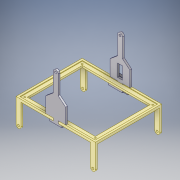
# Autodesk Inventor part: ControllerPCBHolder
Saved by Autodesk Inventor 2019.1 (Build 231200000, 200)
## iProperties
Created: 2018-09-15
Part Number: ControllerPCBHolder
Material: Generisch
Document SubType Name: Modeling
Designer: JochenAlt
Density: 1 g/cm^3
Appearance: Nylon 6
Author: JochenAlt
Autodesk Inventor part; units mm, degrees
ref_plane "YZ Plane" through (0, 0, 0) normal (1, 0, 0) x (0, 1, 0)
ref_plane "XZ Plane" through (0, 0, 0) normal (0, 1, 0) x (-1, 0, 0)
ref_plane "XY Plane" through (0, 0, 0) normal (0, 0, 1) x (1, 0, 0)
sketch "Skizze1" plane through (0, 0, 0) normal (0, 0, 1) x (1, 0, 0)
  line L0 (-61, 50.5) -> (61, 50.5)
  line L1 (61, 50.5) -> (61, -50.5)
  line L2 (61, -50.5) -> (-61, -50.5)
  line L3 (-61, -50.5) -> (-61, 50.5)
  line L4 (0, 70.7) -> (0, -70.7) construction
  line L5 (-85.4, 0) -> (85.4, 0) construction
  line L6 (-55, 44.5) -> (55, 44.5)
  line L7 (55, 44.5) -> (55, -44.5)
  line L8 (55, -44.5) -> (-55, -44.5)
  line L9 (-55, -44.5) -> (-55, 44.5)
  line L10 (-57.15, 46.36) -> (57.15, 46.36) construction
  line L11 (57.15, 46.36) -> (57.15, -46.36) construction
  line L12 (57.15, -46.36) -> (-57.15, -46.36) construction
  line L13 (-57.15, -46.36) -> (-57.15, 46.36) construction
  circle A0 centre (-57.15, 46.36) radius 1.25
  circle A1 centre (57.15, 46.36) radius 1.25
  circle A2 centre (-57.15, -46.36) radius 1.25
  circle A3 centre (57.15, -46.36) radius 1.25
  point P0 (0, 0)
  dimension "d0" = 122
  dimension "d1" = 101
  dimension "d4" = 6
  dimension "d5" = 6
  dimension "d6" = 2.5
  dimension "d7" = 114.3
  dimension "d8" = 92.72
  constraints: 24 end point, 6 parallel, 4 centre point, 4 coincident, 3 equal radius, 3 horizontal, 3 perpendicular, 6 other
  measures "d0" distance of L0.start L0.end
  measures "d1" distance of L0.end L1.end
  measures "d4" distance between parallel lines of L6 L0
  measures "d5" distance between parallel lines of L9 L3
  measures "d6" diameter of A0
  measures "d7" distance of L11.end L12.end
  measures "d8" distance of L10.end L11.end
extrude "Extrusion2" add sketch "Skizze1" along normal blind 3
sketch "Skizze2" plane through (0, 0, 0) normal (0, 1, 0) x (-1, 0, 0)
  arc A0 (56.1888, -34.75) -> (64.1888, -34.75) centre (60.1888, -34.75) ccw
  arc A1 (-64.1888, -34.75) -> (-56.1888, -34.75) centre (-60.1888, -34.75) ccw
  line L0 (0, -98.1) -> (0, 102.1) construction
  line L1 (-97.3, 0) -> (97.3, 0) construction
  circle A2 centre (60.1888, -34.75) radius 1.75
  circle A3 centre (-60.1888, -34.75) radius 1.75
  line L2 (64.1888, -34.75) -> (64.1888, 3)
  line L3 (56.1888, -34.75) -> (56.1888, 3)
  line L4 (-56.1888, -34.75) -> (-56.1888, 3)
  line L5 (-64.1888, -34.75) -> (-64.1888, 3)
  line L6 (-61, 3) -> (61, 3) construction
  line L7 (64.1888, 3) -> (56.1888, 3)
  line L8 (-64.1888, 3) -> (-56.1888, 3)
  circle A4 centre (0, 69.5) radius 1.75
  arc A5 (4, 69.5) -> (-4, 69.5) centre (0, 69.5) ccw
  line L9 (60.1888, -34.75) -> (0, 69.5) construction
  line L10 (4, 69.5) -> (4, 39)
  line L11 (-4, 0) -> (-4, 9)
  line L12 (61, 0) -> (-61, 0) projected
  circle A6 centre (0, 0) radius 69.5 construction
  line L13 (60.1888, -34.75) -> (-60.1888, -34.75) construction
  line L14 (0, 69.5) -> (-60.1888, -34.75) construction
  line L15 (-4.15, 0) -> (-4.15, 4)
  line L16 (-4.15, 4) -> (-4, 4)
  line L17 (4.15, 4) -> (4.15, 0)
  line L18 (55, 3) -> (-55, 3) construction
  line L19 (4.15, 0) -> (4, 0)
  line L20 (4, 0) -> (4, 0)
  line L21 (-4, 0) -> (-4.15, 0)
  line L22 (4, 0) -> (-4, 0)
  line L23 (4.15, 4) -> (16, 4)
  line L24 (16, 4) -> (16, 29)
  line L25 (16, 29) -> (4, 39)
  line L26 (4, 39) -> (-4, 39)
  line L27 (-4, 39) -> (-16, 29)
  line L28 (-16, 29) -> (-16, 4)
  line L29 (-16, 4) -> (-4.15, 4)
  line L30 (4, 29) -> (-4, 29)
  line L31 (4, 29) -> (4, 9)
  line L32 (-4, 29) -> (-4, 39)
  line L33 (4, 39) -> (4, 29)
  line L34 (-4, 39) -> (-4, 69.5)
  line L35 (4, 9) -> (-4, 9)
  line L36 (4, 9) -> (4, 4)
  line L37 (-4, 9) -> (-4, 29)
  line L38 (4, 4) -> (4, 0)
  line L39 (-4, 4) -> (4.15, 4)
  dimension "d12" = 3.5
  dimension "d22" = 69.5
  dimension "d23" = 4
  dimension "d42" = 0.15
  dimension "d44" = 1
  dimension "d54" = 25
  dimension "d55" = 10
  dimension "d56" = 12
  dimension "d57" = 5
  constraints: 70 end point, 14 tangent, 13 perpendicular, 9 point on line, 8 point on circle, 7 centre point, 6 horizontal, 6 vertical, 4 equal radius, 3 coincident, 3 equal length, 1 collinear, 3 other
  measures "d12" diameter of A2
  measures "d22" radius of A6
  measures "d23" radius of A0
  measures "d42" distance between parallel lines of L15 L11
  measures "d44" distance between parallel lines of L18 L16
  measures "d54" distance of L23.end L24.end
  measures "d55" vertical distance of L10.end L24.end
  measures "d56" horizontal distance of L10.end L24.end
  measures "d57" distance between parallel lines of L35 L16
extrude "Extrusion3" add sketch "Skizze2" along normal blind 3 from surface at 50.5 contours L3 L7 L2 A0 | L5 L8 L4 A1
extrude "Extrusion4" add sketch "Skizze2" against normal blind 3 from surface at -50.5 contours L3 L7 L2 A0 | L5 L8 L4 A1
sketch "Skizze4" plane through (0, 0, 0) normal (0, 0, 1) x (1, 0, 0)
  line L0 (-64.1888, 53.5) -> (-64.1888, 50.5) projected
  line L1 (56.1888, -53.5) -> (64.1888, -53.5) projected
  line L2 (-64.1888, 53.5) -> (64.1888, 53.5)
  line L3 (64.1888, 53.5) -> (64.1888, -53.5)
  line L4 (64.1888, -53.5) -> (-64.1888, -53.5)
  line L5 (-64.1888, -53.5) -> (-64.1888, 53.5)
  line L6 (61, -50.5) -> (61, 50.5) projected
  line L7 (61, -50.5) -> (-61, -50.5)
  line L8 (-61, -50.5) -> (-61, 50.5)
  line L9 (-61, 50.5) -> (61, 50.5)
  line L10 (61, 50.5) -> (61, -50.5)
  point P0 (0, 0)
  constraints: 16 end point, 4 parallel, 2 horizontal, 2 perpendicular, 1 coincident
extrude "Extrusion5" add sketch "Skizze4" along normal blind 4
extrude "Extrusion7" cut sketch "Skizze2" along normal up to surface (3 mm away) from surface at -53.5 contours L17 L12 L38 L39 | L38 L12 L11 L39
extrude "Extrusion8" cut sketch "Skizze2" against normal up to surface (3 mm away) from surface at 53.5 contours L17 L12 L38 L39 | L38 L12 L11 L39
sketch "Skizze5" plane through (0, 0, 0) normal (0, 1, 0) x (-1, 0, 0)
  point P0 (0, 0)
sketch "Skizze6" plane through (-56.1888, 53.5, 0) normal (0, -1, 0) x (1, 0, 0)
  line L0 (-33.6755, 0) -> (146.053, 0) construction
  line L1 (56.1888, 19.15) -> (56.1888, -48.4) construction
  line L2 (45.1888, 7.5) -> (64.1888, 7.5)
  line L3 (64.1888, 7.5) -> (64.1888, -8.5)
  line L4 (64.1888, -8.5) -> (45.1888, -8.5)
  line L5 (45.1888, -8.5) -> (45.1888, 7.5)
  line L6 (112.3775, 0) -> (0, 0) projected
  circle A0 centre (47.6888, -6) radius 1.75
  circle A1 centre (61.6888, -6) radius 1.75
  line L7 (61.6888, -6) -> (47.6888, -6) construction
  line L8 (54.6888, 7.5) -> (54.6888, -8.5) construction
  line L9 (43.1888, -10.5) -> (66.1888, -10.5)
  line L10 (66.1888, -10.5) -> (66.1888, 9.5)
  line L11 (66.1888, 9.5) -> (43.1888, 9.5)
  line L12 (43.1888, 9.5) -> (43.1888, -10.5)
  point P0 (56.1888, 0)
  point P1 (56.1888, 0)
  point P2 (56.1888, 0)
  dimension "d24" = 19
  dimension "d25" = 16
  dimension "d29" = 7.5
  dimension "d30" = 3.5
  dimension "d31" = 2.5
  dimension "d32" = 14
  dimension "d33" = 8
  dimension "d48" = 2
  constraints: 20 end point, 4 parallel, 3 midpoint, 3 perpendicular, 2 centre point, 2 horizontal, 1 coincident, 1 equal radius, 1 symmetric about line, 4 other
  measures "d24" distance of L3.end L4.end
  measures "d25" distance of L2.end L3.end
  measures "d29" distance from line of L2 point (56.189, 0)
  measures "d30" diameter of A0
  measures "d31" distance from line of L4 L7.start
  measures "d32" distance of L7.start L7.end
  measures "d33" distance between parallel lines of L3 L1
  measures "d48" distance between parallel lines of L4 L9
extrude "Extrusion6" add sketch "Skizze2" against normal up to surface (3 mm away) from surface at -50.5 separate body contours L10 L26 L34 A5 | L33 L30 L32 L26 | L25 L24 L23 L39 L36 L31 L33 | L32 L37 L11 L16 L29 L28 L27 | L31 L35 L37 L30 | L36 L39 L11 L35 | L17 L12 L38 L39 | L38 L12 L11 L39 | L16 L11 L12 L15
extrude "Extrusion9" add sketch "Skizze2" against normal up to surface (3 mm away) from surface at 53.5 contours L10 L26 L34 A5 | L33 L30 L32 L26 | L25 L24 L23 L39 L36 L31 L33 | L32 L37 L11 L16 L29 L28 L27 | L36 L39 L11 L35 | L17 L12 L38 L39 | L38 L12 L11 L39 | L16 L11 L12 L15 bodies 2
sketch "Skizze7" plane through (4, -53.5, 0) normal (0, 0, -1) x (-1, 0, 0)
  line L0 (-52.1888, 0) -> (60.1888, 0) construction
  line L1 (17, 0) -> (14, 0)
  line L2 (-6, 0) -> (-6, 9)
  line L3 (-6, 9) -> (14, 9)
  line L4 (17, 9) -> (17, 0)
  line L5 (59, 9) -> (-51, 9) construction
  line L6 (17, 107) -> (-6, 107)
  line L7 (-6, 107) -> (-6, 98)
  line L8 (-6, 98) -> (17, 98)
  line L9 (17, 98) -> (17, 107)
  line L10 (59, 98) -> (-51, 98) projected
  line L11 (-60.1888, 107) -> (68.1888, 107) projected
  line L12 (8, 3) -> (8, 0) construction
  line L13 (0, 3) -> (0, 0) construction
  line L14 (2.25, 3) -> (5.75, 3) construction
  line L15 (2.25, 0) -> (5.75, 0) construction
  line L16 (8.15, 3) -> (0, 3) construction
  line L17 (4, 3) -> (4, 0) construction
  line L18 (8, 0) -> (0, 0) construction
  line L19 (14, 9) -> (14, 0)
  line L20 (14, 9) -> (17, 9)
  line L21 (14, 0) -> (-6, 0)
  point P0 (4, 53.5)
  point P1 (8.15, 0)
  point P2 (-0.15, 107)
  point P3 (-0.15, 3)
  dimension "d45" = 23
  dimension "d51" = 10
  constraints: 24 end point, 7 parallel, 5 point on line, 3 horizontal, 3 perpendicular, 2 collinear, 1 midpoint, 1 other
  measures "d45" distance between parallel lines of L2 L4
  measures "d51" distance between parallel lines of L17 L2
extrude "Extrusion10" add sketch "Skizze7" along normal blind 3 contours L9 L8 L7 L6 bodies 2
extrude "Extrusion12" add sketch "Skizze7" along normal blind 3 contours L21 L2 L3 L19 bodies 2
extrude "Extrusion11" add sketch "Skizze6" against normal blind 4 bodies 2
equation "\"d5\" = d4"
equation "\"d44\" = d43"
equation "\"d43\" = 1"
